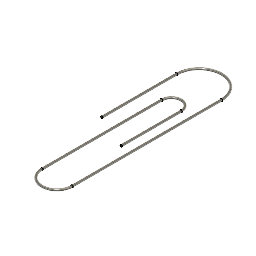
safety pins (Autodesk Fusion 360 design; units mm, degrees)
part number: 2025-11-30-20-20-52-722
Autodesk Fusion 360 part; units mm, degrees
sketch "Sketch1" plane through (0, 0, 0) normal (0, 1, 0) x (1, 0, 0)
  line L0 (0, 0) -> (0, 50)
  line L1 (0, 50) -> (30, 50) construction
  line L2 (30, 50) -> (30, -50)
  line L3 (30, -50) -> (10, -50) construction
  line L4 (10, -50) -> (10, 30)
  line L5 (10, 30) -> (23, 30) construction
  line L6 (23, 30) -> (23, -10)
  line L7 (23, -10) -> (17, -10) construction
  arc A0 (30, 50) -> (0, 50) centre (15, 50) ccw
  arc A1 (23, 30) -> (10, 30) centre (16.5, 30) ccw
  arc A2 (10, -50) -> (30, -50) centre (20, -50) ccw
  dimension "d1" = 50
  dimension "d2" = 30
  dimension "d3" = 100
  dimension "d4" = 20
  dimension "d5" = 80
  dimension "d6" = 13
  dimension "d7" = 6
  dimension "d8" = 40
  dimension "d9" = 7
  dimension "d10" = 15
  constraint coincident L0.start origin
  constraint vertical L0
  constraint perpendicular L0 L1
  constraint perpendicular L1 L2
  constraint perpendicular L2 L3
  constraint perpendicular L3 L4
  constraint perpendicular L4 L5
  constraint perpendicular L5 L6
  constraint perpendicular L6 L7
  constraint coincident L1 L2.start
  constraint tangent L0 A0
  constraint tangent L4 A1
  constraint tangent L4 A2
  measures "d1" distance of L0.start L0.end
  measures "d2" distance of L0.end L1.end
  measures "d3" distance of L1.end L2.end
  measures "d4" distance of L2.end L3.end
  measures "d5" distance of L3.end L4.end
  measures "d6" distance of L4.end L5.end
  measures "d7" distance of L6.end L7.end
  measures "d8" distance of L5.end L6.end
  measures "d9" distance of L2 L6.end
  measures "d10" radius of A0
sketch "Sketch2" plane through (0, 0, 0) normal (0, 0, 1) x (1, 0, 0)
  circle A0 centre (0, 0) radius 0.75
  dimension "d11" = 1.5
  constraint coincident A0.centre origin
  measures "d11" diameter of A0
sweep "Sweep1" add profiles "Sketch2" path "Sketch1" along L0 A0 L2 A2 L4 A1 L6 section 1
